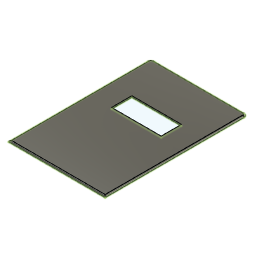
HuCard Riser (Autodesk Fusion 360 design; units mm, degrees)
Autodesk Fusion 360 part; units mm, degrees
sketch "Sketch1" plane through (0, 0, 0) normal (0, 0, 1) x (1, 0, 0)
  line L0 (52.245, -0.0032) -> (1.8763, -0.0032)
  spline S0 degree 3 poles (1.8763, -0.0032) (0.841, -0.0032) (0.0018, -0.8424) (0.0018, -1.8778) knots 0 0 0 0 1 1 1 1
  line L1 (0.0018, -1.8778) -> (0.0018, -79.8036)
  line L2 (0.0018, -79.8036) -> (54.1196, -79.8036)
  line L3 (54.1196, -79.8036) -> (54.1196, -1.8778)
  spline S1 degree 3 poles (54.1196, -1.8778) (54.1196, -0.8424) (53.2804, -0.0032) (52.245, -0.0032) knots 0 0 0 0 1 1 1 1
  line L4 (40.6841, -34.9282) -> (12.8563, -34.9282)
  line L5 (12.8563, -34.9282) -> (12.8563, -23.5656)
  line L6 (12.8563, -23.5656) -> (40.6841, -23.5656)
  line L7 (40.6841, -23.5656) -> (40.6841, -34.9282)
extrude "Extrude1" add sketch "Sketch1" along normal blind 0.75
extrude "Extrude2" [suppressed]
fillet "Fillet1" radius 0.75 6 edges at (54.1196, -40.8407, 0.75) (53.5706, -0.5522, 0.75) (27.0607, -0.0032, 0.75) (0.5508, -0.5522, 0.75) (0.0018, -40.8407, 0.75) (27.0607, -79.8036, 0.75)
equation "d9 = 2.25 mm - 1.5 mm"
equation "d14 = d9"
named bodies: "HuCard riser"
